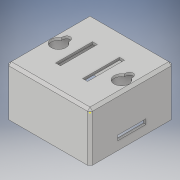
# Autodesk Inventor part: BundOtta
Saved by Autodesk Inventor 2019.1 (Build 231200000, 200)
## iProperties
Created: 2019-08-01
Part Number: BundOtta
Material: Genérico
Document SubType Name: Modeling
Designer: IEEE UFABC
Density: 1 g/cm^3
Appearance: Padrão
Author: IEEE UFABC
Autodesk Inventor part; units mm, degrees
ref_plane "YZ Plane" through (0, 0, 0) normal (1, 0, 0) x (0, 1, 0)
ref_plane "XZ Plane" through (0, 0, 0) normal (0, 1, 0) x (-1, 0, 0)
ref_plane "XY Plane" through (0, 0, 0) normal (0, 0, 1) x (1, 0, 0)
sketch "Esboço1" plane through (0, 0, 0) normal (0, 1, 0) x (-1, 0, 0)
  line L0 (0, 0) -> (68, 0)
  line L1 (68, 0) -> (68, -68)
  line L2 (68, -68) -> (0, -68)
  line L3 (0, -68) -> (0, 0)
  line L4 (66, -2) -> (2, -2)
  line L5 (2, -2) -> (2, -66)
  line L6 (2, -66) -> (66, -66)
  line L7 (66, -66) -> (66, -2)
  dimension "d0" = 68
  dimension "d1" = 68
  dimension "d2" = 2
  dimension "d3" = 2
  dimension "d4" = 2
  dimension "d5" = 2
  constraints: 16 end point, 4 parallel, 2 horizontal, 2 perpendicular
  measures "d0" distance of L1.end L2.end
  measures "d1" distance of L0.end L1.end
  measures "d2" distance between parallel lines of L1 L7
  measures "d3" distance between parallel lines of L6 L2
  measures "d4" distance between parallel lines of L3 L5
  measures "d5" distance between parallel lines of L0 L4
extrude "Extrusão1" add sketch "Esboço1" along normal blind 38
sketch "Esboço2" plane through (0, 38, 0) normal (0, 1, 0) x (1, 0, 0)
  line L0 (-68, 68) -> (0, 68) projected
  line L1 (0, 0) -> (-68, 0)
  line L2 (-68, 0) -> (-68, 68)
  line L3 (-68, 68) -> (0, 68)
  line L4 (0, 68) -> (0, 0)
  constraints: 8 end point, 2 parallel, 1 horizontal, 1 perpendicular
extrude "Extrusão2" add sketch "Esboço2" along normal blind 2
chamfer "Chanfro1" distance 2 angle 45 8 edges at (-68, 20, -68) (0, 20, -68) (-68, 20, 0) (0, 20, 0) (0, 40, -34) (-34, 40, -68) (-68, 40, -34) (-34, 40, 0)
sketch "Esboço3" plane through (0, 0, -2) normal (1, 0, 0) x (0, 0, -1)
  line L0 (64, 0) -> (0, 0) construction
  line L1 (32, 11) -> (32, 0) construction
  line L2 (43.5, 11) -> (20.5, 11)
  line L3 (20.5, 11) -> (20.5, 7)
  line L4 (20.5, 7) -> (43.5, 7)
  line L5 (43.5, 7) -> (43.5, 11)
  point P0 (-2, 0)
  dimension "d16" = 4
  dimension "d17" = 11
  dimension "d18" = 23
  constraints: 10 end point, 2 parallel, 1 horizontal, 1 midpoint, 1 perpendicular
  measures "d16" distance of L3.end L2.end
  measures "d17" distance between parallel lines of L0 L2
  measures "d18" distance between parallel lines of L3 L5
extrude "Extrusão3" cut sketch "Esboço3" against normal blind 4
sketch "Esboço4" plane through (-68, 0, -66) normal (-1, 0, 0) x (0, 0, 1)
  line L0 (43.5, 11) -> (20.5, 11) projected
  line L1 (43.5, 7) -> (20.5, 7)
  line L2 (20.5, 7) -> (20.5, 11)
  line L3 (20.5, 11) -> (43.5, 11)
  line L4 (43.5, 11) -> (43.5, 7)
  point P0 (66, 0)
  constraints: 8 end point, 2 parallel, 1 horizontal, 1 perpendicular
extrude "Extrusão4" cut sketch "Esboço4" against normal blind 4
sketch "Esboço5" plane through (0, 40, 0) normal (0, 1, 0) x (1, 0, 0)
  line L0 (-34, 66) -> (-34, 2) construction
  line L1 (-43, 49) -> (-47, 49)
  line L2 (-47, 49) -> (-47, 19)
  line L3 (-47, 19) -> (-43, 19)
  line L4 (-43, 19) -> (-43, 49)
  line L5 (-43, 34) -> (-61.5633, 34) construction
  line L6 (-66, 2) -> (-66, 66) construction
  arc A0 (-62.5279, 39.2371) -> (-56.6721, 39.2371) centre (-59.6, 34) ccw
  ellipse E0 centre (-59.6, 40) end of major axis (-56.6, 40) minor radius 3.5 (-56.6721, 39.2371) -> (-62.5279, 39.2371) ccw
  line L7 (-25, 49) -> (-21, 49)
  line L8 (-21, 49) -> (-21, 19)
  line L9 (-21, 19) -> (-25, 19)
  line L10 (-25, 19) -> (-25, 49)
  arc A1 (-11.3279, 39.2371) -> (-5.4721, 39.2371) centre (-8.4, 34) ccw
  ellipse E1 centre (-8.4, 40) end of major axis (-11.4, 40) minor radius 3.5 (-5.4721, 39.2371) -> (-11.3279, 39.2371) ccw
  point P0 (0, 0)
  dimension "d28" = 3
  dimension "d29" = 3.5
  dimension "d23" = 4
  dimension "d24" = 30
  dimension "d25" = 19
  dimension "d26" = 12
  dimension "d27" = 6.4
  constraints: 20 end point, 8 symmetric about line, 6 point on circle, 2 centre point, 2 horizontal, 2 parallel, 1 midpoint, 1 perpendicular, 1 point on line, 1 vertical, 10 other
  measures "d23" distance of L3.end L2.end
  measures "d24" distance of L2.end L1.end
  measures "d26" diameter of A0
extrude "Extrusão5" cut sketch "Esboço5" against normal blind 4
sketch "Esboço6" plane through (0, 38, 0) normal (0, -1, 0) x (1, 0, 0)
  point P0 (0, 0)
sketch "Esboço7" plane through (0, 38, 0) normal (0, -1, 0) x (1, 0, 0)
  line L0 (-15, -2) -> (-17, -2)
  line L1 (-17, -2) -> (-17, -66)
  line L2 (-17, -66) -> (-15, -66)
  line L3 (-15, -66) -> (-15, -2)
  line L4 (-2, -2) -> (-2, -66) projected
  line L5 (-34, -66) -> (-34, -2) construction
  line L6 (-15, -2) -> (-17, -2) construction
  line L7 (-15, -2) -> (-17, -2)
  line L8 (-53, -2) -> (-51, -2)
  line L9 (-51, -2) -> (-51, -66)
  line L10 (-51, -66) -> (-53, -66)
  line L11 (-53, -66) -> (-53, -2)
  point P0 (0, 0)
  dimension "d32" = 2
  dimension "d33" = 13
  constraints: 22 end point, 4 symmetric about line, 2 parallel, 1 horizontal, 1 perpendicular
  measures "d32" distance of L2.end L1.end
  measures "d33" distance between parallel lines of L4 L3
extrude "Extrusão6" add sketch "Esboço7" along normal blind 14
